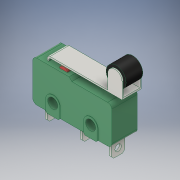
# Autodesk Inventor part: MSW-13
Saved by Autodesk Inventor 2019 (Build 230136000, 136)
## iProperties
Created: 2021-01-03
Part Number: MSW-13
Material: Пластик АБС
Document SubType Name: Modeling
Designer: Professional
Density: 1.06 g/cm^3
Appearance: Гладкий — темный цвет морской волны
Author: Professional
Autodesk Inventor part; units mm, degrees
ref_plane "YZ Plane" through (0, 0, 0) normal (1, 0, 0) x (0, 1, 0)
ref_plane "XZ Plane" through (0, 0, 0) normal (0, 1, 0) x (-1, 0, 0)
ref_plane "XY Plane" through (0, 0, 0) normal (0, 0, 1) x (1, 0, 0)
sketch "Эскиз2" plane through (0, 0, 0) normal (0, 0, 1) x (1, 0, 0)
  line L0 (1, 0) -> (18.8, 0)
  line L1 (19.8, 1) -> (19.8, 8.5)
  line L2 (18.8, 9.5) -> (9.8, 9.5)
  line L3 (9.8, 9.5) -> (9.1, 10.2)
  line L4 (9.1, 10.2) -> (1, 10.2)
  line L5 (0, 9.2) -> (0, 1)
  arc A0 (1, 10.2) -> (0, 9.2) centre (1, 9.2) ccw
  arc A1 (0, 1) -> (1, 0) centre (1, 1) ccw
  arc A2 (18.8, 0) -> (19.8, 1) centre (18.8, 1) ccw
  arc A3 (19.8, 8.5) -> (18.8, 9.5) centre (18.8, 8.5) ccw
  point P0 (0, 0)
  point P1 (19.8, 0)
  point P2 (19.8, 9.5)
  dimension "d42" = 19.8
  dimension "d43" = 9.5
  dimension "d44" = 10
  dimension "d45" = 135
  dimension "d46" = 10.2
  dimension "d47" = 1
  constraints: 12 end point, 8 point on circle, 8 tangent, 6 point on line, 4 centre point, 3 equal radius, 3 perpendicular, 1 horizontal, 1 parallel
  measures "d42" distance of point (0, 0) point (19.8, 0)
  measures "d43" distance of point (19.8, 0) point (19.8, 9.5)
  measures "d44" distance of point (19.8, 9.5) L2.end
  measures "d45" angle of L2 L3
  measures "d46" distance between parallel lines of L4 L0
  measures "d47" radius of A0
extrude "Выдавливание1" add sketch "Эскиз2" along normal mid plane 6.4
sketch "Эскиз3" plane through (0, 0, 0) normal (0, 0, 1) x (1, 0, 0)
  line L0 (1, 0) -> (18.8, 0) projected
  line L1 (1.6, 0) -> (2.1, 0)
  line L2 (2.1, 0) -> (2.1, -4)
  line L3 (2.1, -4) -> (1.6, -4)
  line L4 (1.6, -4) -> (1.6, 0)
  line L5 (10.4, 0) -> (10.9, 0)
  line L6 (10.9, 0) -> (10.9, -4)
  line L7 (10.9, -4) -> (10.4, -4)
  line L8 (10.4, -4) -> (10.4, 0)
  line L9 (17.7, 0) -> (18.2, 0)
  line L10 (18.2, 0) -> (18.2, -4)
  line L11 (18.2, -4) -> (17.7, -4)
  line L12 (17.7, -4) -> (17.7, 0)
  line L13 (0, 9.2) -> (0, 1) projected
  point P0 (0, 0)
  point P1 (1.85, -4)
  point P2 (17.95, -4)
  point P3 (10.65, -4)
  dimension "d51" = 0.5
  dimension "d52" = 8.8
  dimension "d53" = 7.3
  dimension "d54" = 4
  dimension "d55" = 1.85
  constraints: 24 end point, 6 parallel, 4 point on line, 3 horizontal, 3 midpoint, 3 perpendicular, 2 collinear, 1 horizontal alignment
  measures "d51" distance between parallel lines of L2 L4
  measures "d52" distance of point (1.85, -4) point (10.65, -4)
  measures "d53" distance of point (17.95, -4) point (10.65, -4)
  measures "d54" distance from line of L0 point (17.95, -4)
  measures "d55" distance from line of L13 point (1.85, -4)
extrude "Выдавливание2" add sketch "Эскиз3" along normal mid plane 3.4
sketch "Эскиз4" plane through (0, 0, 0) normal (0, 0, 1) x (1, 0, 0)
  arc A0 (6.9, 2.5) -> (3.3, 2.5) centre (5.1, 2.5) ccw
  line L0 (3.3, 2.5) -> (3.3, 0)
  line L1 (18.8, 0) -> (1, 0) projected
  line L2 (3.3, 0) -> (3.7, -0.4)
  line L3 (3.7, -0.4) -> (6.5, -0.4)
  line L4 (6.5, -0.4) -> (6.9, 0)
  line L5 (6.9, 0) -> (6.9, 2.5)
  line L6 (12.8, 0) -> (13.2, -0.4)
  line L7 (13.2, -0.4) -> (16, -0.4)
  line L8 (16, -0.4) -> (16.4, 0)
  line L9 (16.4, 0) -> (16.4, 2.5)
  line L10 (12.8, 0) -> (12.8, 2.5)
  arc A1 (16.4, 2.5) -> (12.8, 2.5) centre (14.6, 2.5) ccw
  line L11 (0, 1) -> (0, 9.2) projected
  point P0 (0, 0)
  dimension "d58" = 0.4
  dimension "d59" = 2.5
  dimension "d60" = 1.8
  dimension "d61" = 135
  dimension "d62" = 9.5
  dimension "d63" = 5.1
  constraints: 20 end point, 4 equal length, 4 perpendicular, 4 point on circle, 4 tangent, 3 point on line, 2 centre point, 2 vertical, 1 equal radius, 1 horizontal, 1 horizontal alignment
  measures "d58" distance between parallel lines of L3 L1
  measures "d59" distance from line of L1 A0.centre
  measures "d60" radius of A0
  measures "d61" angle of L8 L7
  measures "d62" distance of A0.centre A1.centre
  measures "d63" distance from line of L11 A0.centre
extrude "Выдавливание3" add sketch "Эскиз4" along normal mid plane 6.6
sketch "Эскиз6" plane through (0, 0, 3.3) normal (0, 0, 1) x (1, 0, 0)
  arc A0 (6.9, 2.5) -> (3.3, 2.5) centre (5.1, 2.5) ccw projected
  arc A1 (16.4, 2.5) -> (12.8, 2.5) centre (14.6, 2.5) ccw projected
  point P0 (0, 0)
  constraints: 2 coincident
hole "Отверстие1" at (5.1, 2.5, 3.3) at (14.6, 2.5, 3.3) direction (0, 0, -1) diameter 2.5 end through all
sketch "Эскиз7" plane through (0, 0, 0) normal (0, 0, 1) x (1, 0, 0)
  line L0 (1, 10.2) -> (9.1, 10.2) projected
  line L1 (2.8, 10.2) -> (2.8, 10.7)
  line L2 (3.5, 11.4) -> (18, 11.4)
  line L3 (18, 11.4) -> (18, 15)
  line L4 (21.6, 15) -> (21.6, 11)
  line L5 (21.6, 11) -> (3.7, 11)
  line L6 (3.2, 10.5) -> (3.2, 10.2)
  arc A0 (21.6, 15) -> (18, 15) centre (19.8, 15) ccw
  line L7 (0, 9.2) -> (0, 1) projected
  arc A1 (3.7, 11) -> (3.2, 10.5) centre (3.7, 10.5) ccw
  arc A2 (3.5, 11.4) -> (2.8, 10.7) centre (3.5, 10.7) ccw
  point P0 (0, 0)
  point P1 (2.8, 11.4)
  point P2 (3.2, 11)
  dimension "d73" = 0.4
  dimension "d74" = 2.8
  dimension "d75" = 17
  dimension "d76" = 1.8
  dimension "d77" = 0.4
  dimension "d78" = 0.8
  dimension "d79" = 4
  dimension "d82" = 0.5
  dimension "d83" = 0.7
  constraints: 12 end point, 6 point on circle, 6 point on line, 6 tangent, 3 centre point, 3 perpendicular, 2 vertical, 1 parallel
  measures "d73" distance between parallel lines of L2 L5
  measures "d74" distance between parallel lines of L7 L1
  measures "d75" distance from line of A0.centre L1
  measures "d76" radius of A0
  measures "d77" distance between parallel lines of L1 L6
  measures "d78" distance between parallel lines of L0 L5
  measures "d79" distance from line of L5 A0.centre
  measures "d82" radius of A1
  measures "d83" radius of A2
extrude "Выдавливание4" add sketch "Эскиз7" along normal mid plane 4.8
sketch "Эскиз8" plane through (0, 0, 0) normal (0, 0, 1) x (1, 0, 0)
  line L0 (3.5, 11.4) -> (18, 11.4) projected
  line L1 (9.8542, 11.4) -> (26.7526, 11.4)
  line L2 (26.7526, 11.4) -> (26.7526, 19.641)
  line L3 (26.7526, 19.641) -> (9.8542, 19.641)
  line L4 (9.8542, 19.641) -> (9.8542, 11.4)
  point P0 (0, 0)
  point P1 (19.8, 15)
  constraints: 8 end point, 2 parallel, 1 horizontal, 1 perpendicular, 1 point on line
extrude "Выдавливание5" cut sketch "Эскиз8" along normal mid plane 4.2
sketch "Эскиз9" plane through (0, 0, 0) normal (0, 0, 1) x (1, 0, 0)
  arc A0 (21.6, 15) -> (18, 15) centre (19.8, 15) ccw projected
  circle A1 centre (19.8, 15) radius 2.5
  point P0 (0, 0)
  dimension "d87" = 5
  constraints: 1 centre point, 1 coincident
  measures "d87" diameter of A1
extrude "Выдавливание6" add sketch "Эскиз9" along normal mid plane 4.2
sketch "Эскиз10" plane through (1.6, -4, 1.7) normal (-1, 0, 0) x (0, 0, 1)
  circle A0 centre (-1.7, 1.7) radius 0.8
  line L0 (-3.4, 0) -> (0, 0) projected
  point P0 (-1.7, 4)
  dimension "d90" = 1.6
  dimension "d91" = 1.7
  constraints: 1 centre point
  measures "d90" diameter of A0
  measures "d91" distance from line of L0 A0.centre
extrude "Выдавливание7" cut sketch "Эскиз10" against normal through all
chamfer "Фаска1" distance 0.6 angle 45 6 edges at (1.85, -4, -1.7) (10.65, -4, -1.7) (17.95, -4, -1.7) (10.65, -4, 1.7) (1.85, -4, 1.7) (17.95, -4, 1.7)
sketch "Эскиз11" plane through (0, 0, 0) normal (0, 0, 1) x (1, 0, 0)
  arc A0 (8, 10.4633) -> (6, 10.4633) centre (7, 9.8) ccw
  line L0 (6, 10.4633) -> (6, 10.2)
  line L1 (6, 10.2) -> (8, 10.2)
  line L2 (9.1, 10.2) -> (1, 10.2) projected
  line L3 (8, 10.4633) -> (8, 10.2)
  line L4 (3.7, 11) -> (21.6, 11) projected
  line L5 (0, 9.2) -> (0, 1) projected
  point P0 (0, 0)
  dimension "d97" = 1.2
  dimension "d98" = 2
  dimension "d99" = 6
  constraints: 6 end point, 2 point on circle, 1 centre point, 1 horizontal, 1 horizontal alignment, 1 parallel, 1 perpendicular, 1 point on line, 1 tangent, 1 vertical
  measures "d97" radius of A0
  measures "d98" distance between parallel lines of L3 L0
  measures "d99" distance between parallel lines of L5 L0
extrude "Выдавливание8" add sketch "Эскиз11" along normal mid plane 5
